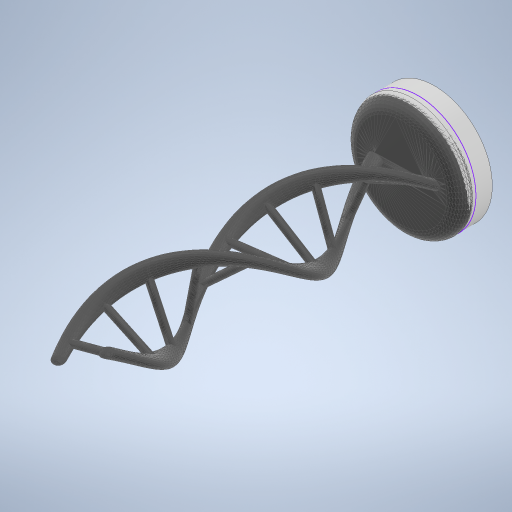
# Autodesk Inventor part: Double Helix DNA
Saved by Autodesk Inventor 2024.2 (Build 282272000, 272)
## iProperties
Created: 2025-11-29
Part Number: Double Helix DNA
Material: Типовые
Document SubType Name: Modeling
Designer: Zakhar
Density: 1 g/cm^3
Appearance: По умолчанию
Author: Zakhar
Autodesk Inventor part; units mm, degrees
ref_plane "YZ Plane" through (0, 0, 0) normal (1, 0, 0) x (0, 1, 0)
ref_plane "XZ Plane" through (0, 0, 0) normal (0, 1, 0) x (-1, 0, 0)
ref_plane "XY Plane" through (0, 0, 0) normal (0, 0, 1) x (1, 0, 0)
sketch "Эскиз1" plane through (-5.2498, 5.9143, 126.7955) normal (0, 0, -1) x (-1, 0, 0)
  circle A0 centre (-11.6693, 11.6262) radius 34.7667
  point P0 (-5.2498, -5.9143)
  constraints: 1 centre point
extrude "Выдавливание1" add sketch "Эскиз1" along normal blind 10 and the other way blind 7
fillet "Сопряжение1" radius 4 1 edges at (41.1862, 17.5406, 133.7955)
sketch "Эскиз3" plane through (6.4195, 17.5406, 116.7955) normal (0, 0, -1) x (-1, 0, 0)
  line L0 (-31.3596, 4.1297) -> (-9.5444, 4.1297) construction
  line L1 (-9.5444, 4.1297) -> (-9.5444, 1.0806) construction
  line L2 (-9.5444, 1.0806) -> (-31.3596, 1.0806) construction
  line L3 (-31.3596, 1.0806) -> (-31.3596, 4.1297) construction
  line L4 (-30.1606, 1.7317) -> (-29.7609, 1.7317)
  line L5 (-29.7609, 1.7317) -> (-29.7609, 2.531)
  spline S0 degree 2 poles (-29.7609, 2.531) (-29.7609, 3.2038) (-28.8283, 4.1297) (-28.1622, 4.1297) knots 0 0 0 1 2 2 2
  line L6 (-28.1622, 4.1297) -> (-27.7626, 4.1297)
  spline S1 degree 2 poles (-27.7626, 4.1297) (-27.3629, 4.1297) (-27.3629, 3.73) knots 0 0 0 1 1 1
  spline S2 degree 2 poles (-27.3629, 3.73) (-27.3629, 3.3303) (-27.7626, 3.3303) knots 0 0 0 1 1 1
  line L7 (-27.7626, 3.3303) -> (-28.1622, 3.3303)
  spline S3 degree 2 poles (-28.1622, 3.3303) (-28.4953, 3.3303) (-28.9616, 2.864) (-28.9616, 2.531) knots 0 0 0 1 2 2 2
  line L8 (-28.9616, 2.531) -> (-28.9616, 1.7317)
  line L9 (-28.9616, 1.7317) -> (-27.7626, 1.7317)
  spline S4 degree 2 poles (-27.7626, 1.7317) (-27.3629, 1.7317) (-27.3629, 1.332) knots 0 0 0 1 1 1
  spline S5 degree 2 poles (-27.3629, 1.332) (-27.3629, 0.9323) (-27.7626, 0.9323) knots 0 0 0 1 1 1
  line L10 (-27.7626, 0.9323) -> (-28.9616, 0.9323)
  line L11 (-28.9616, 0.9323) -> (-28.9616, -3.4707)
  spline S6 degree 2 poles (-28.9616, -3.4707) (-28.9616, -3.8703) (-29.3612, -3.8703) knots 0 0 0 1 1 1
  spline S7 degree 2 poles (-29.3612, -3.8703) (-29.7609, -3.8703) (-29.7609, -3.4707) knots 0 0 0 1 1 1
  line L12 (-29.7609, -3.4707) -> (-29.7609, 0.9323)
  line L13 (-29.7609, 0.9323) -> (-30.1606, 0.9323)
  spline S8 degree 2 poles (-30.1606, 0.9323) (-30.5602, 0.9323) (-30.5602, 1.332) knots 0 0 0 1 1 1
  spline S9 degree 2 poles (-30.5602, 1.332) (-30.5602, 1.7317) (-30.1606, 1.7317) knots 0 0 0 1 1 1
  spline S10 degree 2 poles (-25.7576, 3.73) (-25.7576, 4.1297) (-25.3579, 4.1297) knots 0 0 0 1 1 1
  spline S11 degree 2 poles (-25.3579, 4.1297) (-24.9582, 4.1297) (-24.9582, 3.73) knots 0 0 0 1 1 1
  line L14 (-24.9582, 3.73) -> (-24.9582, -2.6713)
  spline S12 degree 2 poles (-24.9582, -2.6713) (-24.9582, -2.9778) (-24.1589, -3.1643) (-24.1589, -3.4707) knots 0 0 0 1 2 2 2
  spline S13 degree 2 poles (-24.1589, -3.4707) (-24.1589, -3.8703) (-24.5586, -3.8703) knots 0 0 0 1 1 1
  spline S14 degree 2 poles (-24.5586, -3.8703) (-25.0981, -3.8703) (-25.7576, -3.2309) (-25.7576, -2.6713) knots 0 0 0 1 2 2 2
  line L15 (-25.7576, -2.6713) -> (-25.7576, 3.73)
  line L16 (-22.1539, 1.7317) -> (-21.7542, 1.7317)
  line L17 (-21.7542, 1.7317) -> (-21.7542, 2.531)
  spline S15 degree 2 poles (-21.7542, 2.531) (-21.7542, 3.2038) (-20.8217, 4.1297) (-20.1556, 4.1297) knots 0 0 0 1 2 2 2
  line L18 (-20.1556, 4.1297) -> (-19.7559, 4.1297)
  spline S16 degree 2 poles (-19.7559, 4.1297) (-19.3562, 4.1297) (-19.3562, 3.73) knots 0 0 0 1 1 1
  spline S17 degree 2 poles (-19.3562, 3.73) (-19.3562, 3.3303) (-19.7559, 3.3303) knots 0 0 0 1 1 1
  line L19 (-19.7559, 3.3303) -> (-20.1556, 3.3303)
  spline S18 degree 2 poles (-20.1556, 3.3303) (-20.4886, 3.3303) (-20.9549, 2.864) (-20.9549, 2.531) knots 0 0 0 1 2 2 2
  line L20 (-20.9549, 2.531) -> (-20.9549, 1.7317)
  line L21 (-20.9549, 1.7317) -> (-19.7559, 1.7317)
  spline S19 degree 2 poles (-19.7559, 1.7317) (-19.3562, 1.7317) (-19.3562, 1.332) knots 0 0 0 1 1 1
  spline S20 degree 2 poles (-19.3562, 1.332) (-19.3562, 0.9323) (-19.7559, 0.9323) knots 0 0 0 1 1 1
  line L22 (-19.7559, 0.9323) -> (-20.9549, 0.9323)
  line L23 (-20.9549, 0.9323) -> (-20.9549, -3.4707)
  spline S21 degree 2 poles (-20.9549, -3.4707) (-20.9549, -3.8703) (-21.3546, -3.8703) knots 0 0 0 1 1 1
  spline S22 degree 2 poles (-21.3546, -3.8703) (-21.7542, -3.8703) (-21.7542, -3.4707) knots 0 0 0 1 1 1
  line L24 (-21.7542, -3.4707) -> (-21.7542, 0.9323)
  line L25 (-21.7542, 0.9323) -> (-22.1539, 0.9323)
  spline S23 degree 2 poles (-22.1539, 0.9323) (-22.5536, 0.9323) (-22.5536, 1.332) knots 0 0 0 1 1 1
  spline S24 degree 2 poles (-22.5536, 1.332) (-22.5536, 1.7317) (-22.1539, 1.7317) knots 0 0 0 1 1 1
  line L26 (-16.9516, -1.2725) -> (-16.9516, -3.4707)
  spline S25 degree 2 poles (-16.9516, -3.4707) (-16.9516, -3.8703) (-17.3512, -3.8703) knots 0 0 0 1 1 1
  spline S26 degree 2 poles (-17.3512, -3.8703) (-17.7509, -3.8703) (-17.7509, -3.4707) knots 0 0 0 1 1 1
  line L27 (-17.7509, -3.4707) -> (-17.7509, 3.73)
  spline S27 degree 2 poles (-17.7509, 3.73) (-17.7509, 4.1297) (-17.3512, 4.1297) knots 0 0 0 1 1 1
  spline S28 degree 2 poles (-17.3512, 4.1297) (-16.9516, 4.1297) (-16.9516, 3.73) knots 0 0 0 1 1 1
  line L28 (-16.9516, 3.73) -> (-16.9516, -0.2667)
  line L29 (-16.9516, -0.2667) -> (-14.3937, 1.6517)
  spline S29 degree 2 poles (-14.3937, 1.6517) (-14.2871, 1.7317) (-14.1539, 1.7317) knots 0 0 0 1 1 1
  spline S30 degree 2 poles (-14.1539, 1.7317) (-13.7542, 1.7317) (-13.7542, 1.332) knots 0 0 0 1 1 1
  spline S31 degree 2 poles (-13.7542, 1.332) (-13.7542, 1.1255) (-13.9074, 1.0056) knots 0 0 0 1 1 1
  line L30 (-13.9074, 1.0056) -> (-15.4595, -0.1534)
  line L31 (-15.4595, -0.1534) -> (-13.7942, -3.2842)
  spline S32 degree 2 poles (-13.7942, -3.2842) (-13.7542, -3.3641) (-13.7542, -3.4707) knots 0 0 0 1 1 1
  spline S33 degree 2 poles (-13.7542, -3.4707) (-13.7542, -3.6372) (-13.9874, -3.8703) (-14.1539, -3.8703) knots 0 0 0 1 2 2 2
  spline S34 degree 2 poles (-14.1539, -3.8703) (-14.387, -3.8703) (-14.5003, -3.6572) knots 0 0 0 1 1 1
  line L32 (-14.5003, -3.6572) -> (-16.1123, -0.6464)
  line L33 (-16.1123, -0.6464) -> (-16.9516, -1.2725)
  line L34 (-11.7492, 1.7317) -> (-11.3496, 1.7317)
  line L35 (-11.3496, 1.7317) -> (-11.3496, 2.531)
  spline S35 degree 2 poles (-11.3496, 2.531) (-11.3496, 3.2038) (-10.417, 4.1297) (-9.7509, 4.1297) knots 0 0 0 1 2 2 2
  line L36 (-9.7509, 4.1297) -> (-9.3512, 4.1297)
  spline S36 degree 2 poles (-9.3512, 4.1297) (-8.9516, 4.1297) (-8.9516, 3.73) knots 0 0 0 1 1 1
  spline S37 degree 2 poles (-8.9516, 3.73) (-8.9516, 3.3303) (-9.3512, 3.3303) knots 0 0 0 1 1 1
  line L37 (-9.3512, 3.3303) -> (-9.7509, 3.3303)
  spline S38 degree 2 poles (-9.7509, 3.3303) (-10.084, 3.3303) (-10.5502, 2.864) (-10.5502, 2.531) knots 0 0 0 1 2 2 2
  line L38 (-10.5502, 2.531) -> (-10.5502, 1.7317)
  line L39 (-10.5502, 1.7317) -> (-9.3512, 1.7317)
  spline S39 degree 2 poles (-9.3512, 1.7317) (-8.9516, 1.7317) (-8.9516, 1.332) knots 0 0 0 1 1 1
  spline S40 degree 2 poles (-8.9516, 1.332) (-8.9516, 0.9323) (-9.3512, 0.9323) knots 0 0 0 1 1 1
  line L40 (-9.3512, 0.9323) -> (-10.5502, 0.9323)
  line L41 (-10.5502, 0.9323) -> (-10.5502, -3.4707)
  spline S41 degree 2 poles (-10.5502, -3.4707) (-10.5502, -3.8703) (-10.9499, -3.8703) knots 0 0 0 1 1 1
  spline S42 degree 2 poles (-10.9499, -3.8703) (-11.3496, -3.8703) (-11.3496, -3.4707) knots 0 0 0 1 1 1
  line L42 (-11.3496, -3.4707) -> (-11.3496, 0.9323)
  line L43 (-11.3496, 0.9323) -> (-11.7492, 0.9323)
  spline S43 degree 2 poles (-11.7492, 0.9323) (-12.1489, 0.9323) (-12.1489, 1.332) knots 0 0 0 1 1 1
  spline S44 degree 2 poles (-12.1489, 1.332) (-12.1489, 1.7317) (-11.7492, 1.7317) knots 0 0 0 1 1 1
  spline S45 degree 2 poles (-7.3462, 3.73) (-7.3462, 4.1297) (-6.9466, 4.1297) knots 0 0 0 1 1 1
  spline S46 degree 2 poles (-6.9466, 4.1297) (-6.5469, 4.1297) (-6.5469, 3.73) knots 0 0 0 1 1 1
  line L44 (-6.5469, 3.73) -> (-6.5469, -2.6713)
  spline S47 degree 2 poles (-6.5469, -2.6713) (-6.5469, -2.9778) (-5.7476, -3.1643) (-5.7476, -3.4707) knots 0 0 0 1 2 2 2
  spline S48 degree 2 poles (-5.7476, -3.4707) (-5.7476, -3.8703) (-6.1472, -3.8703) knots 0 0 0 1 1 1
  spline S49 degree 2 poles (-6.1472, -3.8703) (-6.6868, -3.8703) (-7.3462, -3.2309) (-7.3462, -2.6713) knots 0 0 0 1 2 2 2
  line L45 (-7.3462, -2.6713) -> (-7.3462, 3.73)
  spline S50 degree 2 poles (-4.1422, 1.332) (-4.1422, 1.7317) (-3.7426, 1.7317) knots 0 0 0 1 1 1
  line L46 (-3.7426, 1.7317) -> (-1.3446, 1.7317)
  spline S51 degree 2 poles (-1.3446, 1.7317) (-0.9449, 1.7317) (-0.9449, 1.332) knots 0 0 0 1 1 1
  line L47 (-0.9449, 1.332) -> (-0.9449, 0.5327)
  spline S52 degree 2 poles (-0.9449, 0.5327) (-0.9449, 0.133) (-1.3446, 0.133) knots 0 0 0 1 1 1
  spline S53 degree 2 poles (-1.3446, 0.133) (-1.7442, 0.133) (-1.7442, 0.5327) knots 0 0 0 1 1 1
  line L48 (-1.7442, 0.5327) -> (-1.7442, 0.9323)
  line L49 (-1.7442, 0.9323) -> (-3.3429, 0.9323)
  line L50 (-3.3429, 0.9323) -> (-3.3429, -3.4707)
  spline S54 degree 2 poles (-3.3429, -3.4707) (-3.3429, -3.8703) (-3.7426, -3.8703) knots 0 0 0 1 1 1
  spline S55 degree 2 poles (-3.7426, -3.8703) (-4.1422, -3.8703) (-4.1422, -3.4707) knots 0 0 0 1 1 1
  line L51 (-4.1422, -3.4707) -> (-4.1422, 1.332)
  line L52 (1.4598, 0.9323) -> (1.0601, 0.9323)
  spline S56 degree 2 poles (1.0601, 0.9323) (0.6604, 0.9323) (0.6604, 1.332) knots 0 0 0 1 1 1
  spline S57 degree 2 poles (0.6604, 1.332) (0.6604, 1.7317) (1.0601, 1.7317) knots 0 0 0 1 1 1
  line L53 (1.0601, 1.7317) -> (1.4598, 1.7317)
  line L54 (1.4598, 1.7317) -> (1.4598, 3.73)
  spline S58 degree 2 poles (1.4598, 3.73) (1.4598, 4.1297) (1.8594, 4.1297) knots 0 0 0 1 1 1
  spline S59 degree 2 poles (1.8594, 4.1297) (2.2591, 4.1297) (2.2591, 3.73) knots 0 0 0 1 1 1
  line L55 (2.2591, 3.73) -> (2.2591, 1.7317)
  line L56 (2.2591, 1.7317) -> (3.4581, 1.7317)
  spline S60 degree 2 poles (3.4581, 1.7317) (3.8578, 1.7317) (3.8578, 1.332) knots 0 0 0 1 1 1
  spline S61 degree 2 poles (3.8578, 1.332) (3.8578, 0.9323) (3.4581, 0.9323) knots 0 0 0 1 1 1
  line L57 (3.4581, 0.9323) -> (2.2591, 0.9323)
  line L58 (2.2591, 0.9323) -> (2.2591, -3.4707)
  spline S62 degree 2 poles (2.2591, -3.4707) (2.2591, -3.8703) (1.8594, -3.8703) knots 0 0 0 1 1 1
  spline S63 degree 2 poles (1.8594, -3.8703) (1.4598, -3.8703) (1.4598, -3.4707) knots 0 0 0 1 1 1
  line L59 (1.4598, -3.4707) -> (1.4598, 0.9323)
  spline S64 degree 2 poles (13.0634, -5.8687) (13.0634, -6.2683) (12.6638, -6.2683) knots 0 0 0 1 1 1
  line L60 (12.6638, -6.2683) -> (3.8644, -6.2683)
  spline S65 degree 2 poles (3.8644, -6.2683) (3.4648, -6.2683) (3.4648, -5.8687) knots 0 0 0 1 1 1
  spline S66 degree 2 poles (3.4648, -5.8687) (3.4648, -5.469) (3.8644, -5.469) knots 0 0 0 1 1 1
  line L61 (3.8644, -5.469) -> (12.6638, -5.469)
  spline S67 degree 2 poles (12.6638, -5.469) (13.0634, -5.469) (13.0634, -5.8687) knots 0 0 0 1 1 1
  line L62 (17.4664, 3.73) -> (17.4664, -1.4723)
  spline S68 degree 2 poles (17.4664, -1.4723) (17.4664, -2.4648) (16.0609, -3.8703) (15.0684, -3.8703) knots 0 0 0 1 2 2 2
  spline S69 degree 2 poles (15.0684, -3.8703) (14.0693, -3.8703) (12.6638, -2.4648) (12.6638, -1.4723) knots 0 0 0 1 2 2 2
  line L63 (12.6638, -1.4723) -> (12.6638, 3.73)
  spline S70 degree 2 poles (12.6638, 3.73) (12.6638, 4.1297) (13.0634, 4.1297) knots 0 0 0 1 1 1
  spline S71 degree 2 poles (13.0634, 4.1297) (13.4631, 4.1297) (13.4631, 3.73) knots 0 0 0 1 1 1
  line L64 (13.4631, 3.73) -> (13.4631, -1.4723)
  spline S72 degree 2 poles (13.4631, -1.4723) (13.4631, -2.1451) (14.389, -3.071) (15.0684, -3.071) knots 0 0 0 1 2 2 2
  spline S73 degree 2 poles (15.0684, -3.071) (15.7412, -3.071) (16.6671, -2.1451) (16.6671, -1.4723) knots 0 0 0 1 2 2 2
  line L65 (16.6671, -1.4723) -> (16.6671, 3.73)
  spline S74 degree 2 poles (16.6671, 3.73) (16.6671, 4.1297) (17.0668, 4.1297) knots 0 0 0 1 1 1
  spline S75 degree 2 poles (17.0668, 4.1297) (17.4664, 4.1297) (17.4664, 3.73) knots 0 0 0 1 1 1
  spline S76 degree 2 poles (23.0684, -3.8703) (22.7887, -3.8703) (22.6821, -3.5773) knots 0 0 0 1 1 1
  line L66 (22.6821, -3.5773) -> (21.8694, -1.4057)
  line L67 (21.8694, -1.4057) -> (21.0568, -3.5639)
  spline S77 degree 2 poles (21.0568, -3.5639) (20.9369, -3.8703) (20.6638, -3.8703) knots 0 0 0 1 1 1
  spline S78 degree 2 poles (20.6638, -3.8703) (20.3507, -3.8703) (20.2574, -3.4973) knots 0 0 0 1 1 1
  line L68 (20.2574, -3.4973) -> (19.0784, 1.2321)
  spline S79 degree 2 poles (19.0784, 1.2321) (19.0651, 1.2854) (19.0651, 1.352) knots 0 0 0 1 1 1
  spline S80 degree 2 poles (19.0651, 1.352) (19.0651, 1.7317) (19.4648, 1.7317) knots 0 0 0 1 1 1
  spline S81 degree 2 poles (19.4648, 1.7317) (19.7845, 1.7317) (19.8511, 1.4252) knots 0 0 0 1 1 1
  line L69 (19.8511, 1.4252) -> (20.737, -2.1185)
  line L70 (20.737, -2.1185) -> (21.4831, -0.1268)
  spline S82 degree 2 poles (21.4831, -0.1268) (21.583, 0.133) (21.8694, 0.133) knots 0 0 0 1 1 1
  spline S83 degree 2 poles (21.8694, 0.133) (22.1425, 0.133) (22.2424, -0.1268) knots 0 0 0 1 1 1
  line L71 (22.2424, -0.1268) -> (22.9885, -2.1251)
  line L72 (22.9885, -2.1251) -> (23.8811, 1.4252)
  spline S84 degree 2 poles (23.8811, 1.4252) (23.961, 1.7317) (24.2674, 1.7317) knots 0 0 0 1 1 1
  spline S85 degree 2 poles (24.2674, 1.7317) (24.4273, 1.7317) (24.6671, 1.5052) (24.6671, 1.352) knots 0 0 0 1 2 2 2
  spline S86 degree 2 poles (24.6671, 1.352) (24.6671, 1.2854) (24.6538, 1.2321) knots 0 0 0 1 1 1
  line L73 (24.6538, 1.2321) -> (23.4681, -3.5173)
  spline S87 degree 2 poles (23.4681, -3.5173) (23.3815, -3.8703) (23.0684, -3.8703) knots 0 0 0 1 1 1
  line L74 (31.0684, 3.73) -> (31.0684, -1.4723)
  spline S88 degree 2 poles (31.0684, -1.4723) (31.0684, -2.4648) (29.6629, -3.8703) (28.6704, -3.8703) knots 0 0 0 1 2 2 2
  spline S89 degree 2 poles (28.6704, -3.8703) (27.6713, -3.8703) (26.2658, -2.4648) (26.2658, -1.4723) knots 0 0 0 1 2 2 2
  line L75 (26.2658, -1.4723) -> (26.2658, 3.73)
  spline S90 degree 2 poles (26.2658, 3.73) (26.2658, 4.1297) (26.6654, 4.1297) knots 0 0 0 1 1 1
  spline S91 degree 2 poles (26.6654, 4.1297) (27.0651, 4.1297) (27.0651, 3.73) knots 0 0 0 1 1 1
  line L76 (27.0651, 3.73) -> (27.0651, -1.4723)
  spline S92 degree 2 poles (27.0651, -1.4723) (27.0651, -2.1451) (27.991, -3.071) (28.6704, -3.071) knots 0 0 0 1 2 2 2
  spline S93 degree 2 poles (28.6704, -3.071) (29.3432, -3.071) (30.2691, -2.1451) (30.2691, -1.4723) knots 0 0 0 1 2 2 2
  line L77 (30.2691, -1.4723) -> (30.2691, 3.73)
  spline S94 degree 2 poles (30.2691, 3.73) (30.2691, 4.1297) (30.6688, 4.1297) knots 0 0 0 1 1 1
  spline S95 degree 2 poles (30.6688, 4.1297) (31.0684, 4.1297) (31.0684, 3.73) knots 0 0 0 1 1 1
  point P0 (6.4195, -17.5406)
  constraints: 2 other
extrude "Выдавливание3" cut sketch "Эскиз3" against normal blind 3
